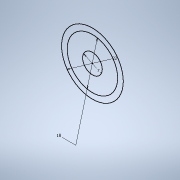
# Autodesk Inventor part: Slip_Ring
Saved by Autodesk Inventor 2022 (Build 260153070, 153G)
## iProperties
Created: 2022-03-05
Part Number: Slip_Ring
Material: Generic
Document SubType Name: Modeling
Designer: a laptop
Density: 1 g/cm^3
Appearance: Default
Author: a laptop
Autodesk Inventor part; units mm, degrees
ref_plane "YZ Plane" through (0, 0, 0) normal (1, 0, 0) x (0, 1, 0)
ref_plane "XZ Plane" through (0, 0, 0) normal (0, 1, 0) x (-1, 0, 0)
ref_plane "XY Plane" through (0, 0, 0) normal (0, 0, 1) x (1, 0, 0)
sketch "Sketch1" plane through (0, 0, 0) normal (0, 0, 1) x (1, 0, 0)
  circle A0 centre (0, 0) radius 9
  circle A1 centre (0, 0) radius 3.5
  circle A2 centre (0, 0) radius 11
  dimension "d0" = 22
  dimension "d1" = 18
  dimension "d2" = 7
  constraints: 3 centre point, 3 coincident
  measures "d0" diameter of A2
  measures "d1" diameter of A0
  measures "d2" diameter of A1
extrude "Extrusion1" add sketch "Sketch1" along normal blind 15.7 contours A2
extrude "Extrusion2" add sketch "Sketch1" along normal blind 16.8 contours A0
body "Solid1"
